Autodesk Fusion 360 part; units mm, degrees
(part 3 of 4)
  line L349 (-93.5315, -46.7348) -> (-93.5315, -40.9333)
  line L350 (-93.5315, -40.9333) -> (-94.3309, -40.9333)
  line L351 (-94.3309, -40.9333) -> (-94.3309, -37.8327)
  line L352 (-94.3309, -37.8327) -> (-93.5315, -37.8327)
  line L353 (-93.5315, -37.8327) -> (-93.5315, -36.8336)
  line L354 (-93.5315, -36.8336) -> (-79.5322, -36.8336)
  line L355 (-79.5322, -36.8336) -> (-79.5322, -37.8327)
  line L356 (-79.5322, -37.8327) -> (-78.7314, -37.8327)
  line L357 (-78.7314, -37.8327) -> (-78.7314, -40.9333)
  line L358 (-78.7314, -40.9333) -> (-79.5322, -40.9333)
  line L359 (-79.5322, -40.9333) -> (-79.5322, -46.7348)
  line L360 (-79.5322, -46.7348) -> (-78.7314, -46.7348)
  line L361 (-78.7314, -46.7348) -> (-78.7314, -49.8327)
  line L362 (-78.7314, -49.8327) -> (-79.5322, -49.8327)
  line L363 (-79.5322, -49.8327) -> (-79.5322, -50.833)
  line L364 (-98.5822, -50.833) -> (-112.5815, -50.833)
  line L365 (-112.5815, -50.833) -> (-112.5815, -49.8327)
  line L366 (-112.5815, -49.8327) -> (-113.3809, -49.8327)
  line L367 (-113.3809, -49.8327) -> (-113.3809, -46.7348)
  line L368 (-113.3809, -46.7348) -> (-112.5815, -46.7348)
  line L369 (-112.5815, -46.7348) -> (-112.5815, -40.9333)
  line L370 (-112.5815, -40.9333) -> (-113.3809, -40.9333)
  line L371 (-113.3809, -40.9333) -> (-113.3809, -37.8327)
  line L372 (-113.3809, -37.8327) -> (-112.5815, -37.8327)
  line L373 (-112.5815, -37.8327) -> (-112.5815, -36.8336)
  line L374 (-112.5815, -36.8336) -> (-98.5822, -36.8336)
  line L375 (-98.5822, -36.8336) -> (-98.5822, -37.8327)
  line L376 (-98.5822, -37.8327) -> (-97.7814, -37.8327)
  line L377 (-97.7814, -37.8327) -> (-97.7814, -40.9333)
  line L378 (-97.7814, -40.9333) -> (-98.5822, -40.9333)
  line L379 (-98.5822, -40.9333) -> (-98.5822, -46.7348)
  line L380 (-98.5822, -46.7348) -> (-97.7814, -46.7348)
  line L381 (-97.7814, -46.7348) -> (-97.7814, -49.8327)
  line L382 (-97.7814, -49.8327) -> (-98.5822, -49.8327)
  line L383 (-98.5822, -49.8327) -> (-98.5822, -50.833)
  line L384 (-227.17, -107.9831) -> (-241.169, -107.9831)
  line L385 (-241.169, -107.9831) -> (-241.169, -106.9826)
  line L386 (-241.169, -106.9826) -> (-241.97, -106.9826)
  line L387 (-241.97, -106.9826) -> (-241.97, -103.8834)
  line L388 (-241.97, -103.8834) -> (-241.169, -103.8834)
  line L389 (-241.169, -103.8834) -> (-241.169, -98.0834)
  line L390 (-241.169, -98.0834) -> (-241.97, -98.0834)
  line L391 (-241.97, -98.0834) -> (-241.97, -94.9828)
  line L392 (-241.97, -94.9828) -> (-241.169, -94.9828)
  line L393 (-241.169, -94.9828) -> (-241.169, -93.9838)
  line L394 (-241.169, -93.9838) -> (-227.17, -93.9838)
  line L395 (-227.17, -93.9838) -> (-227.17, -94.9828)
  line L396 (-227.17, -94.9828) -> (-226.369, -94.9828)
  line L397 (-226.369, -94.9828) -> (-226.369, -98.0834)
  line L398 (-226.369, -98.0834) -> (-227.17, -98.0834)
  line L399 (-227.17, -98.0834) -> (-227.17, -103.8834)
  line L400 (-227.17, -103.8834) -> (-226.369, -103.8834)
  line L401 (-226.369, -103.8834) -> (-226.369, -106.9826)
  line L402 (-226.369, -106.9826) -> (-227.17, -106.9826)
  line L403 (-227.17, -106.9826) -> (-227.17, -107.9831)
  line L404 (-193.832, -50.833) -> (-207.832, -50.833)
  line L405 (-207.832, -50.833) -> (-207.832, -49.8327)
  line L406 (-207.832, -49.8327) -> (-208.631, -49.8327)
  line L407 (-208.631, -49.8327) -> (-208.631, -46.7348)
  line L408 (-208.631, -46.7348) -> (-207.832, -46.7348)
  line L409 (-207.832, -46.7348) -> (-207.832, -40.9333)
  line L410 (-207.832, -40.9333) -> (-208.631, -40.9333)
  line L411 (-208.631, -40.9333) -> (-208.631, -37.8327)
  line L412 (-208.631, -37.8327) -> (-207.832, -37.8327)
  line L413 (-207.832, -37.8327) -> (-207.832, -36.8336)
  line L414 (-207.832, -36.8336) -> (-193.832, -36.8336)
  line L415 (-193.832, -36.8336) -> (-193.832, -37.8327)
  line L416 (-193.832, -37.8327) -> (-193.031, -37.8327)
  line L417 (-193.031, -37.8327) -> (-193.031, -40.9333)
  line L418 (-193.031, -40.9333) -> (-193.832, -40.9333)
  line L419 (-193.832, -40.9333) -> (-193.832, -46.7348)
  line L420 (-193.832, -46.7348) -> (-193.031, -46.7348)
  line L421 (-193.031, -46.7348) -> (-193.031, -49.8327)
  line L422 (-193.031, -49.8327) -> (-193.832, -49.8327)
  line L423 (-193.832, -49.8327) -> (-193.832, -50.833)
  line L424 (-65.2447, -88.9331) -> (-79.244, -88.9331)
  line L425 (-79.244, -88.9331) -> (-79.244, -87.9326)
  line L426 (-79.244, -87.9326) -> (-80.0448, -87.9326)
  line L427 (-80.0448, -87.9326) -> (-80.0448, -84.8334)
  line L428 (-80.0448, -84.8334) -> (-79.244, -84.8334)
  line L429 (-79.244, -84.8334) -> (-79.244, -79.0334)
  line L430 (-79.244, -79.0334) -> (-80.0448, -79.0334)
  line L431 (-80.0448, -79.0334) -> (-80.0448, -75.9328)
  line L432 (-80.0448, -75.9328) -> (-79.244, -75.9328)
  line L433 (-79.244, -75.9328) -> (-79.244, -74.9338)
  line L434 (-79.244, -74.9338) -> (-65.2447, -74.9338)
  line L435 (-65.2447, -74.9338) -> (-65.2447, -75.9328)
  line L436 (-65.2447, -75.9328) -> (-64.4439, -75.9328)
  line L437 (-64.4439, -75.9328) -> (-64.4439, -79.0334)
  line L438 (-64.4439, -79.0334) -> (-65.2447, -79.0334)
  line L439 (-65.2447, -79.0334) -> (-65.2447, -84.8334)
  line L440 (-65.2447, -84.8334) -> (-64.4439, -84.8334)
  line L441 (-64.4439, -84.8334) -> (-64.4439, -87.9326)
  line L442 (-64.4439, -87.9326) -> (-65.2447, -87.9326)
  line L443 (-65.2447, -87.9326) -> (-65.2447, -88.9331)
  line L444 (-198.595, -88.9331) -> (-212.594, -88.9331)
  line L445 (-212.594, -88.9331) -> (-212.594, -87.9326)
  line L446 (-212.594, -87.9326) -> (-213.395, -87.9326)
  line L447 (-213.395, -87.9326) -> (-213.395, -84.8334)
  line L448 (-213.395, -84.8334) -> (-212.594, -84.8334)
  line L449 (-212.594, -84.8334) -> (-212.594, -79.0334)
  line L450 (-212.594, -79.0334) -> (-213.395, -79.0334)
  line L451 (-213.395, -79.0334) -> (-213.395, -75.9328)
  line L452 (-213.395, -75.9328) -> (-212.594, -75.9328)
  line L453 (-212.594, -75.9328) -> (-212.594, -74.9338)
  line L454 (-212.594, -74.9338) -> (-198.595, -74.9338)
  line L455 (-198.595, -74.9338) -> (-198.595, -75.9328)
  line L456 (-198.595, -75.9328) -> (-197.794, -75.9328)
  line L457 (-197.794, -75.9328) -> (-197.794, -79.0334)
  line L458 (-197.794, -79.0334) -> (-198.595, -79.0334)
  line L459 (-198.595, -79.0334) -> (-198.595, -84.8334)
  line L460 (-198.595, -84.8334) -> (-197.794, -84.8334)
  line L461 (-197.794, -84.8334) -> (-197.794, -87.9326)
  line L462 (-197.794, -87.9326) -> (-198.595, -87.9326)
  line L463 (-198.595, -87.9326) -> (-198.595, -88.9331)
  line L464 (-222.407, -69.8831) -> (-236.407, -69.8831)
  line L465 (-236.407, -69.8831) -> (-236.407, -68.8826)
  line L466 (-236.407, -68.8826) -> (-237.206, -68.8826)
  line L467 (-237.206, -68.8826) -> (-237.206, -65.7834)
  line L468 (-237.206, -65.7834) -> (-236.407, -65.7834)
  line L469 (-236.407, -65.7834) -> (-236.407, -59.9834)
  line L470 (-236.407, -59.9834) -> (-237.206, -59.9834)
  line L471 (-237.206, -59.9834) -> (-237.206, -56.8828)
  line L472 (-237.206, -56.8828) -> (-236.407, -56.8828)
  line L473 (-236.407, -56.8828) -> (-236.407, -55.8838)
  line L474 (-236.407, -55.8838) -> (-222.407, -55.8838)
  line L475 (-222.407, -55.8838) -> (-222.407, -56.8828)
  line L476 (-222.407, -56.8828) -> (-221.606, -56.8828)
  line L477 (-221.606, -56.8828) -> (-221.606, -59.9834)
  line L478 (-221.606, -59.9834) -> (-222.407, -59.9834)
  line L479 (-222.407, -59.9834) -> (-222.407, -65.7834)
  line L480 (-222.407, -65.7834) -> (-221.606, -65.7834)
  line L481 (-221.606, -65.7834) -> (-221.606, -68.8826)
  line L482 (-221.606, -68.8826) -> (-222.407, -68.8826)
  line L483 (-222.407, -68.8826) -> (-222.407, -69.8831)
  line L484 (-122.395, -88.9331) -> (-136.394, -88.9331)
  line L485 (-136.394, -88.9331) -> (-136.394, -87.9326)
  line L486 (-136.394, -87.9326) -> (-137.195, -87.9326)
  line L487 (-137.195, -87.9326) -> (-137.195, -84.8334)
  line L488 (-137.195, -84.8334) -> (-136.394, -84.8334)
  line L489 (-136.394, -84.8334) -> (-136.394, -79.0334)
  line L490 (-136.394, -79.0334) -> (-137.195, -79.0334)
  line L491 (-137.195, -79.0334) -> (-137.195, -75.9328)
  line L492 (-137.195, -75.9328) -> (-136.394, -75.9328)
  line L493 (-136.394, -75.9328) -> (-136.394, -74.9338)
  line L494 (-136.394, -74.9338) -> (-122.395, -74.9338)
  line L495 (-122.395, -74.9338) -> (-122.395, -75.9328)
  line L496 (-122.395, -75.9328) -> (-121.594, -75.9328)
  line L497 (-121.594, -75.9328) -> (-121.594, -79.0334)
  line L498 (-121.594, -79.0334) -> (-122.395, -79.0334)
  line L499 (-122.395, -79.0334) -> (-122.395, -84.8334)
  line L500 (-122.395, -84.8334) -> (-121.594, -84.8334)
  line L501 (-121.594, -84.8334) -> (-121.594, -87.9326)
  line L502 (-121.594, -87.9326) -> (-122.395, -87.9326)
  line L503 (-122.395, -87.9326) -> (-122.395, -88.9331)
  line L504 (-89.0572, -69.8831) -> (-103.0565, -69.8831)
  line L505 (-103.0565, -69.8831) -> (-103.0565, -68.8826)
  line L506 (-103.0565, -68.8826) -> (-103.8559, -68.8826)
  line L507 (-103.8559, -68.8826) -> (-103.8559, -65.7834)
  line L508 (-103.8559, -65.7834) -> (-103.0565, -65.7834)
  line L509 (-103.0565, -65.7834) -> (-103.0565, -59.9834)
  line L510 (-103.0565, -59.9834) -> (-103.8559, -59.9834)
  line L511 (-103.8559, -59.9834) -> (-103.8559, -56.8828)
  line L512 (-103.8559, -56.8828) -> (-103.0565, -56.8828)
  line L513 (-103.0565, -56.8828) -> (-103.0565, -55.8838)
  line L514 (-103.0565, -55.8838) -> (-89.0572, -55.8838)
  line L515 (-89.0572, -55.8838) -> (-89.0572, -56.8828)
  line L516 (-89.0572, -56.8828) -> (-88.2564, -56.8828)
  line L517 (-88.2564, -56.8828) -> (-88.2564, -59.9834)
  line L518 (-88.2564, -59.9834) -> (-89.0572, -59.9834)
  line L519 (-89.0572, -59.9834) -> (-89.0572, -65.7834)
  line L520 (-89.0572, -65.7834) -> (-88.2564, -65.7834)
  line L521 (-88.2564, -65.7834) -> (-88.2564, -68.8826)
  line L522 (-88.2564, -68.8826) -> (-89.0572, -68.8826)
  line L523 (-89.0572, -68.8826) -> (-89.0572, -69.8831)
  line L524 (-160.495, -88.9331) -> (-174.494, -88.9331)
  line L525 (-174.494, -88.9331) -> (-174.494, -87.9326)
  line L526 (-174.494, -87.9326) -> (-175.295, -87.9326)
  line L527 (-175.295, -87.9326) -> (-175.295, -84.8334)
  line L528 (-175.295, -84.8334) -> (-174.494, -84.8334)
  line L529 (-174.494, -84.8334) -> (-174.494, -79.0334)
  line L530 (-174.494, -79.0334) -> (-175.295, -79.0334)
  line L531 (-175.295, -79.0334) -> (-175.295, -75.9328)
  line L532 (-175.295, -75.9328) -> (-174.494, -75.9328)
  line L533 (-174.494, -75.9328) -> (-174.494, -74.9338)
  line L534 (-174.494, -74.9338) -> (-160.495, -74.9338)
  line L535 (-160.495, -74.9338) -> (-160.495, -75.9328)
  line L536 (-160.495, -75.9328) -> (-159.694, -75.9328)
  line L537 (-159.694, -75.9328) -> (-159.694, -79.0334)
  line L538 (-159.694, -79.0334) -> (-160.495, -79.0334)
  line L539 (-160.495, -79.0334) -> (-160.495, -84.8334)
  line L540 (-160.495, -84.8334) -> (-159.694, -84.8334)
  line L541 (-159.694, -84.8334) -> (-159.694, -87.9326)
  line L542 (-159.694, -87.9326) -> (-160.495, -87.9326)
  line L543 (-160.495, -87.9326) -> (-160.495, -88.9331)
  line L544 (-139.062, -31.7831) -> (-153.063, -31.7831)
  line L545 (-153.063, -31.7831) -> (-153.063, -30.7827)
  line L546 (-153.063, -30.7827) -> (-153.862, -30.7827)
  line L547 (-153.862, -30.7827) -> (-153.862, -27.6848)
  line L548 (-153.862, -27.6848) -> (-153.063, -27.6848)
  line L549 (-153.063, -27.6848) -> (-153.063, -27.0826)
  line L550 (-153.063, -27.0826) -> (-192.687, -27.0826)
  line L551 (-192.687, -27.0826) -> (-192.687, -30.3128)
  line L552 (-192.687, -30.3128) -> (-194.412, -30.3128)
  line L553 (-194.412, -30.3128) -> (-194.412, -31.2347)
  line L554 (-194.412, -31.2347) -> (-197.713, -31.2347)
  line L555 (-197.713, -31.2347) -> (-197.713, -30.3128)
  line L556 (-197.713, -30.3128) -> (-199.438, -30.3128)
  line L557 (-199.438, -30.3128) -> (-199.438, -27.0826)
  line L558 (-199.438, -27.0826) -> (-200.262, -27.0826)
  line L559 (-200.262, -27.0826) -> (-200.262, -24.2838)
  line L560 (-200.262, -24.2838) -> (-199.438, -24.2838)
  line L561 (-199.438, -24.2838) -> (-199.438, -18.0138)
  line L562 (-199.438, -18.0138) -> (-197.713, -18.0138)
  line L563 (-197.713, -18.0138) -> (-197.713, -17.0326)
  line L564 (-197.713, -17.0326) -> (-194.412, -17.0326)
  line L565 (-194.412, -17.0326) -> (-194.412, -18.0138)
  line L566 (-194.412, -18.0138) -> (-192.687, -18.0138)
  line L567 (-192.687, -18.0138) -> (-192.687, -22.4841)
  line L568 (-192.687, -22.4841) -> (-153.063, -22.4841)
  line L569 (-153.063, -22.4841) -> (-153.063, -21.8833)
  line L570 (-153.063, -21.8833) -> (-153.862, -21.8833)
  line L571 (-153.862, -21.8833) -> (-153.862, -18.7827)
  line L572 (-153.862, -18.7827) -> (-153.063, -18.7827)
  line L573 (-153.063, -18.7827) -> (-153.063, -17.7836)
  line L574 (-153.063, -17.7836) -> (-139.062, -17.7836)
  line L575 (-139.062, -17.7836) -> (-139.062, -18.7827)
  line L576 (-139.062, -18.7827) -> (-138.263, -18.7827)
  line L577 (-138.263, -18.7827) -> (-138.263, -21.8833)
  line L578 (-138.263, -21.8833) -> (-139.062, -21.8833)
  line L579 (-139.062, -21.8833) -> (-139.062, -22.4841)
  line L580 (-139.062, -22.4841) -> (-99.4381, -22.4841)
  line L581 (-99.4381, -22.4841) -> (-99.4381, -18.0138)
  line L582 (-99.4381, -18.0138) -> (-97.7126, -18.0138)
  line L583 (-97.7126, -18.0138) -> (-97.7126, -17.0326)
  line L584 (-97.7126, -17.0326) -> (-94.412, -17.0326)
  line L585 (-94.412, -17.0326) -> (-94.412, -18.0138)
  line L586 (-94.412, -18.0138) -> (-92.687, -18.0138)
  line L587 (-92.687, -18.0138) -> (-92.687, -24.2838)
  line L588 (-92.687, -24.2838) -> (-91.8629, -24.2838)
  line L589 (-91.8629, -24.2838) -> (-91.8629, -27.0826)
  line L590 (-91.8629, -27.0826) -> (-92.687, -27.0826)
  line L591 (-92.687, -27.0826) -> (-92.687, -30.3128)
  line L592 (-92.687, -30.3128) -> (-94.412, -30.3128)
  line L593 (-94.412, -30.3128) -> (-94.412, -31.2347)
  line L594 (-94.412, -31.2347) -> (-97.7126, -31.2347)
  line L595 (-97.7126, -31.2347) -> (-97.7126, -30.3128)
  line L596 (-97.7126, -30.3128) -> (-99.4381, -30.3128)
  line L597 (-99.4381, -30.3128) -> (-99.4381, -27.0826)
  line L598 (-99.4381, -27.0826) -> (-139.062, -27.0826)
  line L599 (-139.062, -27.0826) -> (-139.062, -27.6848)
  line L600 (-139.062, -27.6848) -> (-138.263, -27.6848)
  line L601 (-138.263, -27.6848) -> (-138.263, -30.7827)
  line L602 (-138.263, -30.7827) -> (-139.062, -30.7827)
  line L603 (-139.062, -30.7827) -> (-139.062, -31.7831)
  line L604 (-272.412, -69.8831) -> (-286.413, -69.8831)
  line L605 (-286.413, -69.8831) -> (-286.413, -68.8826)
  line L606 (-286.413, -68.8826) -> (-287.212, -68.8826)
  line L607 (-287.212, -68.8826) -> (-287.212, -65.7834)
  line L608 (-287.212, -65.7834) -> (-286.413, -65.7834)
  line L609 (-286.413, -65.7834) -> (-286.413, -65.1826)
  line L610 (-286.413, -65.1826) -> (-287.937, -65.1826)
  line L611 (-287.937, -65.1826) -> (-287.937, -68.4127)
  line L612 (-287.937, -68.4127) -> (-289.662, -68.4127)
  line L613 (-289.662, -68.4127) -> (-289.662, -69.3334)
  line L614 (-289.662, -69.3334) -> (-292.963, -69.3334)
  line L615 (-292.963, -69.3334) -> (-292.963, -68.4127)
  line L616 (-292.963, -68.4127) -> (-294.688, -68.4127)
  line L617 (-294.688, -68.4127) -> (-294.688, -65.1826)
  line L618 (-294.688, -65.1826) -> (-295.512, -65.1826)
  line L619 (-295.512, -65.1826) -> (-295.512, -62.3837)
  line L620 (-295.512, -62.3837) -> (-294.688, -62.3837)
  line L621 (-294.688, -62.3837) -> (-294.688, -56.1138)
  line L622 (-294.688, -56.1138) -> (-292.963, -56.1138)
  line L623 (-292.963, -56.1138) -> (-292.963, -55.1327)
  line L624 (-292.963, -55.1327) -> (-289.662, -55.1327)
  line L625 (-289.662, -55.1327) -> (-289.662, -56.1138)
  line L626 (-289.662, -56.1138) -> (-287.937, -56.1138)
  line L627 (-287.937, -56.1138) -> (-287.937, -60.5828)
  line L628 (-287.937, -60.5828) -> (-286.413, -60.5828)
  line L629 (-286.413, -60.5828) -> (-286.413, -59.9834)
  line L630 (-286.413, -59.9834) -> (-287.212, -59.9834)
  line L631 (-287.212, -59.9834) -> (-287.212, -56.8828)
  line L632 (-287.212, -56.8828) -> (-286.413, -56.8828)
  line L633 (-286.413, -56.8828) -> (-286.413, -55.8838)
  line L634 (-286.413, -55.8838) -> (-272.412, -55.8838)
  line L635 (-272.412, -55.8838) -> (-272.412, -56.8828)
  line L636 (-272.412, -56.8828) -> (-271.611, -56.8828)
  line L637 (-271.611, -56.8828) -> (-271.611, -59.9834)
  line L638 (-271.611, -59.9834) -> (-272.412, -59.9834)
  line L639 (-272.412, -59.9834) -> (-272.412, -60.5828)
  line L640 (-272.412, -60.5828) -> (-270.888, -60.5828)
  line L641 (-270.888, -60.5828) -> (-270.888, -56.1138)
  line L642 (-270.888, -56.1138) -> (-269.161, -56.1138)
  line L643 (-269.161, -56.1138) -> (-269.161, -55.1327)
  line L644 (-269.161, -55.1327) -> (-265.862, -55.1327)
  line L645 (-265.862, -55.1327) -> (-265.862, -56.1138)
  line L646 (-265.862, -56.1138) -> (-264.137, -56.1138)
  line L647 (-264.137, -56.1138) -> (-264.137, -62.3837)
  line L648 (-264.137, -62.3837) -> (-263.313, -62.3837)
  line L649 (-263.313, -62.3837) -> (-263.313, -65.1826)
  line L650 (-263.313, -65.1826) -> (-264.137, -65.1826)
  line L651 (-264.137, -65.1826) -> (-264.137, -68.4127)
  line L652 (-264.137, -68.4127) -> (-265.862, -68.4127)
  line L653 (-265.862, -68.4127) -> (-265.862, -69.3334)
  line L654 (-265.862, -69.3334) -> (-269.161, -69.3334)
  line L655 (-269.161, -69.3334) -> (-269.161, -68.4127)
  line L656 (-269.161, -68.4127) -> (-270.888, -68.4127)
  line L657 (-270.888, -68.4127) -> (-270.888, -65.1826)
  line L658 (-270.888, -65.1826) -> (-272.412, -65.1826)
  line L659 (-272.412, -65.1826) -> (-272.412, -65.7834)
  line L660 (-272.412, -65.7834) -> (-271.611, -65.7834)
  line L661 (-271.611, -65.7834) -> (-271.611, -68.8826)
  line L662 (-271.611, -68.8826) -> (-272.412, -68.8826)
  line L663 (-272.412, -68.8826) -> (-272.412, -69.8831)
  line L664 (-274.795, -107.9831) -> (-288.794, -107.9831)
  line L665 (-288.794, -107.9831) -> (-288.794, -106.9826)
  line L666 (-288.794, -106.9826) -> (-289.595, -106.9826)
  line L667 (-289.595, -106.9826) -> (-289.595, -103.8834)
  line L668 (-289.595, -103.8834) -> (-288.794, -103.8834)
  line L669 (-288.794, -103.8834) -> (-288.794, -103.2826)
  line L670 (-288.794, -103.2826) -> (-290.32, -103.2826)
  line L671 (-290.32, -103.2826) -> (-290.32, -106.5127)
  line L672 (-290.32, -106.5127) -> (-292.045, -106.5127)
  line L673 (-292.045, -106.5127) -> (-292.045, -107.4348)
  line L674 (-292.045, -107.4348) -> (-295.344, -107.4348)
  line L675 (-295.344, -107.4348) -> (-295.344, -106.5127)
  line L676 (-295.344, -106.5127) -> (-297.069, -106.5127)
  line L677 (-297.069, -106.5127) -> (-297.069, -103.2826)
  line L678 (-297.069, -103.2826) -> (-297.895, -103.2826)
  line L679 (-297.895, -103.2826) -> (-297.895, -100.4837)
  line L680 (-297.895, -100.4837) -> (-297.069, -100.4837)
  line L681 (-297.069, -100.4837) -> (-297.069, -94.2138)
  line L682 (-297.069, -94.2138) -> (-295.344, -94.2138)
  line L683 (-295.344, -94.2138) -> (-295.344, -93.2327)
  line L684 (-295.344, -93.2327) -> (-292.045, -93.2327)
  line L685 (-292.045, -93.2327) -> (-292.045, -94.2138)
  line L686 (-292.045, -94.2138) -> (-290.32, -94.2138)
  line L687 (-290.32, -94.2138) -> (-290.32, -98.6828)
  line L688 (-290.32, -98.6828) -> (-288.794, -98.6828)
  line L689 (-288.794, -98.6828) -> (-288.794, -98.0834)
  line L690 (-288.794, -98.0834) -> (-289.595, -98.0834)
  line L691 (-289.595, -98.0834) -> (-289.595, -94.9828)
  line L692 (-289.595, -94.9828) -> (-288.794, -94.9828)
  line L693 (-288.794, -94.9828) -> (-288.794, -93.9838)
  line L694 (-288.794, -93.9838) -> (-274.795, -93.9838)
  line L695 (-274.795, -93.9838) -> (-274.795, -94.9828)
  line L696 (-274.795, -94.9828) -> (-273.994, -94.9828)
  line L697 (-273.994, -94.9828) -> (-273.994, -98.0834)
  line L698 (-273.994, -98.0834) -> (-274.795, -98.0834)
  line L699 (-274.795, -98.0834) -> (-274.795, -98.6828)
  line L700 (-274.795, -98.6828) -> (-273.269, -98.6828)
  line L701 (-273.269, -98.6828) -> (-273.269, -94.2138)
  line L702 (-273.269, -94.2138) -> (-271.544, -94.2138)
  line L703 (-271.544, -94.2138) -> (-271.544, -93.2327)
  line L704 (-271.544, -93.2327) -> (-268.243, -93.2327)
  line L705 (-268.243, -93.2327) -> (-268.243, -94.2138)
  line L706 (-268.243, -94.2138) -> (-266.52, -94.2138)
  line L707 (-266.52, -94.2138) -> (-266.52, -100.4837)
  line L708 (-266.52, -100.4837) -> (-265.694, -100.4837)
  line L709 (-265.694, -100.4837) -> (-265.694, -103.2826)
  line L710 (-265.694, -103.2826) -> (-266.52, -103.2826)
  line L711 (-266.52, -103.2826) -> (-266.52, -106.5127)
  line L712 (-266.52, -106.5127) -> (-268.243, -106.5127)
  line L713 (-268.243, -106.5127) -> (-268.243, -107.4348)
  line L714 (-268.243, -107.4348) -> (-271.544, -107.4348)
  line L715 (-271.544, -107.4348) -> (-271.544, -106.5127)
  line L716 (-271.544, -106.5127) -> (-273.269, -106.5127)
  line L717 (-273.269, -106.5127) -> (-273.269, -103.2826)
  line L718 (-273.269, -103.2826) -> (-274.795, -103.2826)
  line L719 (-274.795, -103.2826) -> (-274.795, -103.8834)
  line L720 (-274.795, -103.8834) -> (-273.994, -103.8834)
  line L721 (-273.994, -103.8834) -> (-273.994, -106.9826)
  line L722 (-273.994, -106.9826) -> (-274.795, -106.9826)
  line L723 (-274.795, -106.9826) -> (-274.795, -107.9831)
  line L724 (-281.937, -31.7831) -> (-295.938, -31.7831)
  line L725 (-295.938, -31.7831) -> (-295.938, -30.7827)
  line L726 (-295.938, -30.7827) -> (-296.737, -30.7827)
  line L727 (-296.737, -30.7827) -> (-296.737, -27.6848)
  line L728 (-296.737, -27.6848) -> (-295.938, -27.6848)
  line L729 (-295.938, -27.6848) -> (-295.938, -21.8833)
  line L730 (-295.938, -21.8833) -> (-296.737, -21.8833)
  line L731 (-296.737, -21.8833) -> (-296.737, -18.7827)
  line L732 (-296.737, -18.7827) -> (-295.938, -18.7827)
  line L733 (-295.938, -18.7827) -> (-295.938, -17.7836)
  line L734 (-295.938, -17.7836) -> (-281.937, -17.7836)
  line L735 (-281.937, -17.7836) -> (-281.937, -18.7827)
  line L736 (-281.937, -18.7827) -> (-281.138, -18.7827)
  line L737 (-281.138, -18.7827) -> (-281.138, -21.8833)
  line L738 (-281.138, -21.8833) -> (-281.937, -21.8833)
  line L739 (-281.937, -21.8833) -> (-281.937, -27.6848)
  line L740 (-281.937, -27.6848) -> (-281.138, -27.6848)
  line L741 (-281.138, -27.6848) -> (-281.138, -30.7827)
  line L742 (-281.138, -30.7827) -> (-281.937, -30.7827)
  line L743 (-281.937, -30.7827) -> (-281.937, -31.7831)
  line L744 (-184.307, -69.8831) -> (-198.307, -69.8831)
  line L745 (-198.307, -69.8831) -> (-198.307, -68.8826)
  line L746 (-198.307, -68.8826) -> (-199.106, -68.8826)
  line L747 (-199.106, -68.8826) -> (-199.106, -65.7834)
  line L748 (-199.106, -65.7834) -> (-198.307, -65.7834)
  line L749 (-198.307, -65.7834) -> (-198.307, -59.9834)
  line L750 (-198.307, -59.9834) -> (-199.106, -59.9834)
  line L751 (-199.106, -59.9834) -> (-199.106, -56.8828)
  line L752 (-199.106, -56.8828) -> (-198.307, -56.8828)
  line L753 (-198.307, -56.8828) -> (-198.307, -55.8838)
  line L754 (-198.307, -55.8838) -> (-184.307, -55.8838)
  line L755 (-184.307, -55.8838) -> (-184.307, -56.8828)
  line L756 (-184.307, -56.8828) -> (-183.506, -56.8828)
  line L757 (-183.506, -56.8828) -> (-183.506, -59.9834)
  line L758 (-183.506, -59.9834) -> (-184.307, -59.9834)
  line L759 (-184.307, -59.9834) -> (-184.307, -65.7834)
  line L760 (-184.307, -65.7834) -> (-183.506, -65.7834)
  line L761 (-183.506, -65.7834) -> (-183.506, -68.8826)
  line L762 (-183.506, -68.8826) -> (-184.307, -68.8826)
  line L763 (-184.307, -68.8826) -> (-184.307, -69.8831)
  line L764 (-217.645, -88.9331) -> (-231.644, -88.9331)
  line L765 (-231.644, -88.9331) -> (-231.644, -87.9326)
  line L766 (-231.644, -87.9326) -> (-232.445, -87.9326)
  line L767 (-232.445, -87.9326) -> (-232.445, -84.8334)
  line L768 (-232.445, -84.8334) -> (-231.644, -84.8334)
  line L769 (-231.644, -84.8334) -> (-231.644, -79.0334)
  line L770 (-231.644, -79.0334) -> (-232.445, -79.0334)
  line L771 (-232.445, -79.0334) -> (-232.445, -75.9328)
  line L772 (-232.445, -75.9328) -> (-231.644, -75.9328)
  line L773 (-231.644, -75.9328) -> (-231.644, -74.9338)
  line L774 (-231.644, -74.9338) -> (-217.645, -74.9338)
  line L775 (-217.645, -74.9338) -> (-217.645, -75.9328)
  line L776 (-217.645, -75.9328) -> (-216.844, -75.9328)
  line L777 (-216.844, -75.9328) -> (-216.844, -79.0334)
  line L778 (-216.844, -79.0334) -> (-217.645, -79.0334)
  line L779 (-217.645, -79.0334) -> (-217.645, -84.8334)
  line L780 (-217.645, -84.8334) -> (-216.844, -84.8334)
  line L781 (-216.844, -84.8334) -> (-216.844, -87.9326)
  line L782 (-216.844, -87.9326) -> (-217.645, -87.9326)
  line L783 (-217.645, -87.9326) -> (-217.645, -88.9331)
  line L784 (-165.257, -69.8831) -> (-179.257, -69.8831)
  line L785 (-179.257, -69.8831) -> (-179.257, -68.8826)
  line L786 (-179.257, -68.8826) -> (-180.056, -68.8826)
  line L787 (-180.056, -68.8826) -> (-180.056, -65.7834)
  line L788 (-180.056, -65.7834) -> (-179.257, -65.7834)
  line L789 (-179.257, -65.7834) -> (-179.257, -59.9834)
  line L790 (-179.257, -59.9834) -> (-180.056, -59.9834)
  line L791 (-180.056, -59.9834) -> (-180.056, -56.8828)
  line L792 (-180.056, -56.8828) -> (-179.257, -56.8828)
  line L793 (-179.257, -56.8828) -> (-179.257, -55.8838)
  line L794 (-179.257, -55.8838) -> (-165.257, -55.8838)
  line L795 (-165.257, -55.8838) -> (-165.257, -56.8828)
  line L796 (-165.257, -56.8828) -> (-164.456, -56.8828)
  line L797 (-164.456, -56.8828) -> (-164.456, -59.9834)
  line L798 (-164.456, -59.9834) -> (-165.257, -59.9834)
  line L799 (-165.257, -59.9834) -> (-165.257, -65.7834)
  line L800 (-165.257, -65.7834) -> (-164.456, -65.7834)
  line L801 (-164.456, -65.7834) -> (-164.456, -68.8826)
  line L802 (-164.456, -68.8826) -> (-165.257, -68.8826)
  line L803 (-165.257, -68.8826) -> (-165.257, -69.8831)
  line L804 (-103.3447, -88.9331) -> (-117.344, -88.9331)
  line L805 (-117.344, -88.9331) -> (-117.344, -87.9326)
  line L806 (-117.344, -87.9326) -> (-118.145, -87.9326)
  line L807 (-118.145, -87.9326) -> (-118.145, -84.8334)
  line L808 (-118.145, -84.8334) -> (-117.344, -84.8334)
  line L809 (-117.344, -84.8334) -> (-117.344, -79.0334)
  line L810 (-117.344, -79.0334) -> (-118.145, -79.0334)
  line L811 (-118.145, -79.0334) -> (-118.145, -75.9328)
  line L812 (-118.145, -75.9328) -> (-117.344, -75.9328)
  line L813 (-117.344, -75.9328) -> (-117.344, -74.9338)
  line L814 (-117.344, -74.9338) -> (-103.3447, -74.9338)
  line L815 (-103.3447, -74.9338) -> (-103.3447, -75.9328)
  line L816 (-103.3447, -75.9328) -> (-102.5439, -75.9328)
  line L817 (-102.5439, -75.9328) -> (-102.5439, -79.0334)
  line L818 (-102.5439, -79.0334) -> (-103.3447, -79.0334)
  line L819 (-103.3447, -79.0334) -> (-103.3447, -84.8334)
  line L820 (-103.3447, -84.8334) -> (-102.5439, -84.8334)
  line L821 (-102.5439, -84.8334) -> (-102.5439, -87.9326)
  line L822 (-102.5439, -87.9326) -> (-103.3447, -87.9326)
  line L823 (-103.3447, -87.9326) -> (-103.3447, -88.9331)
  line L824 (-70.0072, -69.8831) -> (-84.0065, -69.8831)
  line L825 (-84.0065, -69.8831) -> (-84.0065, -68.8826)
  line L826 (-84.0065, -68.8826) -> (-84.8059, -68.8826)
  line L827 (-84.8059, -68.8826) -> (-84.8059, -65.7834)
  line L828 (-84.8059, -65.7834) -> (-84.0065, -65.7834)
  line L829 (-84.0065, -65.7834) -> (-84.0065, -59.9834)
  line L830 (-84.0065, -59.9834) -> (-84.8059, -59.9834)
  line L831 (-84.8059, -59.9834) -> (-84.8059, -56.8828)
  line L832 (-84.8059, -56.8828) -> (-84.0065, -56.8828)
  line L833 (-84.0065, -56.8828) -> (-84.0065, -55.8838)
  line L834 (-84.0065, -55.8838) -> (-70.0072, -55.8838)
  line L835 (-70.0072, -55.8838) -> (-70.0072, -56.8828)
  line L836 (-70.0072, -56.8828) -> (-69.2064, -56.8828)
  line L837 (-69.2064, -56.8828) -> (-69.2064, -59.9834)
  line L838 (-69.2064, -59.9834) -> (-70.0072, -59.9834)
  line L839 (-70.0072, -59.9834) -> (-70.0072, -65.7834)
  line L840 (-70.0072, -65.7834) -> (-69.2064, -65.7834)
  line L841 (-69.2064, -65.7834) -> (-69.2064, -68.8826)
  line L842 (-69.2064, -68.8826) -> (-70.0072, -68.8826)
  line L843 (-70.0072, -68.8826) -> (-70.0072, -69.8831)
  line L844 (-108.1072, -69.8831) -> (-122.107, -69.8831)
  line L845 (-122.107, -69.8831) -> (-122.107, -68.8826)
  line L846 (-122.107, -68.8826) -> (-122.906, -68.8826)
  line L847 (-122.906, -68.8826) -> (-122.906, -65.7834)
  line L848 (-122.906, -65.7834) -> (-122.107, -65.7834)
  line L849 (-122.107, -65.7834) -> (-122.107, -59.9834)
  line L850 (-122.107, -59.9834) -> (-122.906, -59.9834)
  line L851 (-122.906, -59.9834) -> (-122.906, -56.8828)
  line L852 (-122.906, -56.8828) -> (-122.107, -56.8828)
  line L853 (-122.107, -56.8828) -> (-122.107, -55.8838)
  line L854 (-122.107, -55.8838) -> (-108.1072, -55.8838)
  line L855 (-108.1072, -55.8838) -> (-108.1072, -56.8828)
  line L856 (-108.1072, -56.8828) -> (-107.3064, -56.8828)
  line L857 (-107.3064, -56.8828) -> (-107.3064, -59.9834)
  line L858 (-107.3064, -59.9834) -> (-108.1072, -59.9834)
  line L859 (-108.1072, -59.9834) -> (-108.1072, -65.7834)
  line L860 (-108.1072, -65.7834) -> (-107.3064, -65.7834)
  line L861 (-107.3064, -65.7834) -> (-107.3064, -68.8826)
  line L862 (-107.3064, -68.8826) -> (-108.1072, -68.8826)
  line L863 (-108.1072, -68.8826) -> (-108.1072, -69.8831)
  line L864 (-20.0009, -31.7831) -> (-34.0004, -31.7831)
  line L865 (-34.0004, -31.7831) -> (-34.0004, -30.7827)
  line L866 (-34.0004, -30.7827) -> (-34.801, -30.7827)
  line L867 (-34.801, -30.7827) -> (-34.801, -27.6848)
  line L868 (-34.801, -27.6848) -> (-34.0004, -27.6848)
  line L869 (-34.0004, -27.6848) -> (-34.0004, -21.8833)
  line L870 (-34.0004, -21.8833) -> (-34.801, -21.8833)
  line L871 (-34.801, -21.8833) -> (-34.801, -18.7827)
  line L872 (-34.801, -18.7827) -> (-34.0004, -18.7827)
  line L873 (-34.0004, -18.7827) -> (-34.0004, -17.7836)
  line L874 (-34.0004, -17.7836) -> (-20.0009, -17.7836)
  line L875 (-20.0009, -17.7836) -> (-20.0009, -18.7827)
  line L876 (-20.0009, -18.7827) -> (-19.2003, -18.7827)
  line L877 (-19.2003, -18.7827) -> (-19.2003, -21.8833)
  line L878 (-19.2003, -21.8833) -> (-20.0009, -21.8833)
  line L879 (-20.0009, -21.8833) -> (-20.0009, -27.6848)
  line L880 (-20.0009, -27.6848) -> (-19.2003, -27.6848)
  line L881 (-19.2003, -27.6848) -> (-19.2003, -30.7827)
  line L882 (-19.2003, -30.7827) -> (-20.0009, -30.7827)
  line L883 (-20.0009, -30.7827) -> (-20.0009, -31.7831)
  line L884 (-84.2947, -88.9331) -> (-98.294, -88.9331)
  line L885 (-98.294, -88.9331) -> (-98.294, -87.9326)
  line L886 (-98.294, -87.9326) -> (-99.0948, -87.9326)
  line L887 (-99.0948, -87.9326) -> (-99.0948, -84.8334)
  line L888 (-99.0948, -84.8334) -> (-98.294, -84.8334)
  line L889 (-98.294, -84.8334) -> (-98.294, -79.0334)
  line L890 (-98.294, -79.0334) -> (-99.0948, -79.0334)
  line L891 (-99.0948, -79.0334) -> (-99.0948, -75.9328)
  line L892 (-99.0948, -75.9328) -> (-98.294, -75.9328)
  line L893 (-98.294, -75.9328) -> (-98.294, -74.9338)
  line L894 (-98.294, -74.9338) -> (-84.2947, -74.9338)
  line L895 (-84.2947, -74.9338) -> (-84.2947, -75.9328)
  line L896 (-84.2947, -75.9328) -> (-83.4939, -75.9328)
  line L897 (-83.4939, -75.9328) -> (-83.4939, -79.0334)
  line L898 (-83.4939, -79.0334) -> (-84.2947, -79.0334)
  line L899 (-84.2947, -79.0334) -> (-84.2947, -84.8334)
  line L900 (-84.2947, -84.8334) -> (-83.4939, -84.8334)
  line L901 (-83.4939, -84.8334) -> (-83.4939, -87.9326)
  line L902 (-83.4939, -87.9326) -> (-84.2947, -87.9326)
  line L903 (-84.2947, -87.9326) -> (-84.2947, -88.9331)
  line L904 (-46.1947, -88.9331) -> (-60.194, -88.9331)
  line L905 (-60.194, -88.9331) -> (-60.194, -87.9326)
  line L906 (-60.194, -87.9326) -> (-60.9948, -87.9326)
  line L907 (-60.9948, -87.9326) -> (-60.9948, -84.8334)
  line L908 (-60.9948, -84.8334) -> (-60.194, -84.8334)
  line L909 (-60.194, -84.8334) -> (-60.194, -79.0334)
  line L910 (-60.194, -79.0334) -> (-60.9948, -79.0334)
  line L911 (-60.9948, -79.0334) -> (-60.9948, -75.9328)
  line L912 (-60.9948, -75.9328) -> (-60.194, -75.9328)
  line L913 (-60.194, -75.9328) -> (-60.194, -74.9338)
  line L914 (-60.194, -74.9338) -> (-46.1947, -74.9338)
  line L915 (-46.1947, -74.9338) -> (-46.1947, -75.9328)
  line L916 (-46.1947, -75.9328) -> (-45.394, -75.9328)
  line L917 (-45.394, -75.9328) -> (-45.394, -79.0334)
  line L918 (-45.394, -79.0334) -> (-46.1947, -79.0334)
  line L919 (-46.1947, -79.0334) -> (-46.1947, -84.8334)
  line L920 (-46.1947, -84.8334) -> (-45.394, -84.8334)
  line L921 (-45.394, -84.8334) -> (-45.394, -87.9326)
  line L922 (-45.394, -87.9326) -> (-46.1947, -87.9326)
  line L923 (-46.1947, -87.9326) -> (-46.1947, -88.9331)
  line L924 (-212.882, -50.833) -> (-226.882, -50.833)
  line L925 (-226.882, -50.833) -> (-226.882, -49.8327)
  line L926 (-226.882, -49.8327) -> (-227.681, -49.8327)
  line L927 (-227.681, -49.8327) -> (-227.681, -46.7348)
  line L928 (-227.681, -46.7348) -> (-226.882, -46.7348)
  line L929 (-226.882, -46.7348) -> (-226.882, -40.9333)
  line L930 (-226.882, -40.9333) -> (-227.681, -40.9333)
  line L931 (-227.681, -40.9333) -> (-227.681, -37.8327)
  line L932 (-227.681, -37.8327) -> (-226.882, -37.8327)
  line L933 (-226.882, -37.8327) -> (-226.882, -36.8336)
  line L934 (-226.882, -36.8336) -> (-212.882, -36.8336)
  line L935 (-212.882, -36.8336) -> (-212.882, -37.8327)
  line L936 (-212.882, -37.8327) -> (-212.081, -37.8327)
  line L937 (-212.081, -37.8327) -> (-212.081, -40.9333)
  line L938 (-212.081, -40.9333) -> (-212.882, -40.9333)
  line L939 (-212.882, -40.9333) -> (-212.882, -46.7348)
  line L940 (-212.882, -46.7348) -> (-212.081, -46.7348)
  line L941 (-212.081, -46.7348) -> (-212.081, -49.8327)
  line L942 (-212.081, -49.8327) -> (-212.882, -49.8327)
  line L943 (-212.882, -49.8327) -> (-212.882, -50.833)
  line L944 (-136.682, -50.833) -> (-150.682, -50.833)
  line L945 (-150.682, -50.833) -> (-150.682, -49.8327)
  line L946 (-150.682, -49.8327) -> (-151.481, -49.8327)
  line L947 (-151.481, -49.8327) -> (-151.481, -46.7348)
  line L948 (-151.481, -46.7348) -> (-150.682, -46.7348)
  line L949 (-150.682, -46.7348) -> (-150.682, -40.9333)
  line L950 (-150.682, -40.9333) -> (-151.481, -40.9333)
  line L951 (-151.481, -40.9333) -> (-151.481, -37.8327)
  line L952 (-151.481, -37.8327) -> (-150.682, -37.8327)
  line L953 (-150.682, -37.8327) -> (-150.682, -36.8336)
  line L954 (-150.682, -36.8336) -> (-136.682, -36.8336)
  line L955 (-136.682, -36.8336) -> (-136.682, -37.8327)
  line L956 (-136.682, -37.8327) -> (-135.881, -37.8327)
  line L957 (-135.881, -37.8327) -> (-135.881, -40.9333)
  line L958 (-135.881, -40.9333) -> (-136.682, -40.9333)
  line L959 (-136.682, -40.9333) -> (-136.682, -46.7348)
  line L960 (-136.682, -46.7348) -> (-135.881, -46.7348)
  line L961 (-135.881, -46.7348) -> (-135.881, -49.8327)
  line L962 (-135.881, -49.8327) -> (-136.682, -49.8327)
  line L963 (-136.682, -49.8327) -> (-136.682, -50.833)
  line L964 (-117.632, -50.833) -> (-131.632, -50.833)
  line L965 (-131.632, -50.833) -> (-131.632, -49.8327)
  line L966 (-131.632, -49.8327) -> (-132.431, -49.8327)
  line L967 (-132.431, -49.8327) -> (-132.431, -46.7348)
  line L968 (-132.431, -46.7348) -> (-131.632, -46.7348)
  line L969 (-131.632, -46.7348) -> (-131.632, -40.9333)
  line L970 (-131.632, -40.9333) -> (-132.431, -40.9333)
  line L971 (-132.431, -40.9333) -> (-132.431, -37.8327)
  line L972 (-132.431, -37.8327) -> (-131.632, -37.8327)
  line L973 (-131.632, -37.8327) -> (-131.632, -36.8336)
  line L974 (-131.632, -36.8336) -> (-117.632, -36.8336)
  line L975 (-117.632, -36.8336) -> (-117.632, -37.8327)
  line L976 (-117.632, -37.8327) -> (-116.831, -37.8327)
  line L977 (-116.831, -37.8327) -> (-116.831, -40.9333)
  line L978 (-116.831, -40.9333) -> (-117.632, -40.9333)
  line L979 (-117.632, -40.9333) -> (-117.632, -46.7348)
  line L980 (-117.632, -46.7348) -> (-116.831, -46.7348)
  line L981 (-116.831, -46.7348) -> (-116.831, -49.8327)
  line L982 (-116.831, -49.8327) -> (-117.632, -49.8327)
  line L983 (-117.632, -49.8327) -> (-117.632, -50.833)
  line L984 (-208.12, -107.9831) -> (-222.119, -107.9831)
  line L985 (-222.119, -107.9831) -> (-222.119, -106.9826)
  line L986 (-222.119, -106.9826) -> (-222.92, -106.9826)
  line L987 (-222.92, -106.9826) -> (-222.92, -103.8834)
  line L988 (-222.92, -103.8834) -> (-222.119, -103.8834)
  line L989 (-222.119, -103.8834) -> (-222.119, -98.0834)
  line L990 (-222.119, -98.0834) -> (-222.92, -98.0834)
  line L991 (-222.92, -98.0834) -> (-222.92, -94.9828)
  line L992 (-222.92, -94.9828) -> (-222.119, -94.9828)
  line L993 (-222.119, -94.9828) -> (-222.119, -93.9838)
  line L994 (-222.119, -93.9838) -> (-208.12, -93.9838)
  line L995 (-208.12, -93.9838) -> (-208.12, -94.9828)
  line L996 (-208.12, -94.9828) -> (-207.319, -94.9828)
  line L997 (-207.319, -94.9828) -> (-207.319, -98.0834)
  line L998 (-207.319, -98.0834) -> (-208.12, -98.0834)
  line L999 (-208.12, -98.0834) -> (-208.12, -103.8834)
  line L1000 (-208.12, -103.8834) -> (-207.319, -103.8834)
  line L1001 (-207.319, -103.8834) -> (-207.319, -106.9826)
  line L1002 (-207.319, -106.9826) -> (-208.12, -106.9826)
  line L1003 (-208.12, -106.9826) -> (-208.12, -107.9831)
  line L1004 (-60.4822, -50.833) -> (-74.4815, -50.833)
  line L1005 (-74.4815, -50.833) -> (-74.4815, -49.8327)
  line L1006 (-74.4815, -49.8327) -> (-75.2809, -49.8327)
  line L1007 (-75.2809, -49.8327) -> (-75.2809, -46.7348)
  line L1008 (-75.2809, -46.7348) -> (-74.4815, -46.7348)
  line L1009 (-74.4815, -46.7348) -> (-74.4815, -40.9333)
  line L1010 (-74.4815, -40.9333) -> (-75.2809, -40.9333)
  line L1011 (-75.2809, -40.9333) -> (-75.2809, -37.8327)
  line L1012 (-75.2809, -37.8327) -> (-74.4815, -37.8327)
  line L1013 (-74.4815, -37.8327) -> (-74.4815, -36.8336)
  line L1014 (-74.4815, -36.8336) -> (-60.4822, -36.8336)
  line L1015 (-60.4822, -36.8336) -> (-60.4822, -37.8327)
  line L1016 (-60.4822, -37.8327) -> (-59.6814, -37.8327)
  line L1017 (-59.6814, -37.8327) -> (-59.6814, -40.9333)
  line L1018 (-59.6814, -40.9333) -> (-60.4822, -40.9333)
  line L1019 (-60.4822, -40.9333) -> (-60.4822, -46.7348)
  line L1020 (-60.4822, -46.7348) -> (-59.6814, -46.7348)
  line L1021 (-59.6814, -46.7348) -> (-59.6814, -49.8327)
  line L1022 (-59.6814, -49.8327) -> (-60.4822, -49.8327)
  line L1023 (-60.4822, -49.8327) -> (-60.4822, -50.833)
  line L1024 (-189.07, -107.9831) -> (-203.069, -107.9831)
  line L1025 (-203.069, -107.9831) -> (-203.069, -106.9826)
  line L1026 (-203.069, -106.9826) -> (-203.87, -106.9826)
  line L1027 (-203.87, -106.9826) -> (-203.87, -103.8834)
  line L1028 (-203.87, -103.8834) -> (-203.069, -103.8834)
  line L1029 (-203.069, -103.8834) -> (-203.069, -98.0834)
  line L1030 (-203.069, -98.0834) -> (-203.87, -98.0834)
  line L1031 (-203.87, -98.0834) -> (-203.87, -94.9828)
  line L1032 (-203.87, -94.9828) -> (-203.069, -94.9828)
  line L1033 (-203.069, -94.9828) -> (-203.069, -93.9838)
  line L1034 (-203.069, -93.9838) -> (-189.07, -93.9838)
  line L1035 (-189.07, -93.9838) -> (-189.07, -94.9828)
  line L1036 (-189.07, -94.9828) -> (-188.269, -94.9828)
  line L1037 (-188.269, -94.9828) -> (-188.269, -98.0834)
  line L1038 (-188.269, -98.0834) -> (-189.07, -98.0834)
  line L1039 (-189.07, -98.0834) -> (-189.07, -103.8834)
  line L1040 (-189.07, -103.8834) -> (-188.269, -103.8834)
  line L1041 (-188.269, -103.8834) -> (-188.269, -106.9826)
  line L1042 (-188.269, -106.9826) -> (-189.07, -106.9826)
  line L1043 (-189.07, -106.9826) -> (-189.07, -107.9831)
  line L1044 (-246.22, -107.9831) -> (-260.219, -107.9831)
  line L1045 (-260.219, -107.9831) -> (-260.219, -106.9826)
  line L1046 (-260.219, -106.9826) -> (-261.02, -106.9826)
  line L1047 (-261.02, -106.9826) -> (-261.02, -103.8834)
  line L1048 (-261.02, -103.8834) -> (-260.219, -103.8834)
  line L1049 (-260.219, -103.8834) -> (-260.219, -98.0834)
  line L1050 (-260.219, -98.0834) -> (-261.02, -98.0834)
  line L1051 (-261.02, -98.0834) -> (-261.02, -94.9828)
  line L1052 (-261.02, -94.9828) -> (-260.219, -94.9828)
  line L1053 (-260.219, -94.9828) -> (-260.219, -93.9838)
  line L1054 (-260.219, -93.9838) -> (-246.22, -93.9838)
  line L1055 (-246.22, -93.9838) -> (-246.22, -94.9828)
  line L1056 (-246.22, -94.9828) -> (-245.419, -94.9828)
  line L1057 (-245.419, -94.9828) -> (-245.419, -98.0834)
  line L1058 (-245.419, -98.0834) -> (-246.22, -98.0834)
  line L1059 (-246.22, -98.0834) -> (-246.22, -103.8834)
  line L1060 (-246.22, -103.8834) -> (-245.419, -103.8834)
  line L1061 (-245.419, -103.8834) -> (-245.419, -106.9826)
  line L1062 (-245.419, -106.9826) -> (-246.22, -106.9826)
  line L1063 (-246.22, -106.9826) -> (-246.22, -107.9831)
  line L1064 (-241.457, -69.8831) -> (-255.457, -69.8831)
  line L1065 (-255.457, -69.8831) -> (-255.457, -68.8826)
  line L1066 (-255.457, -68.8826) -> (-256.256, -68.8826)
  line L1067 (-256.256, -68.8826) -> (-256.256, -65.7834)
  line L1068 (-256.256, -65.7834) -> (-255.457, -65.7834)
  line L1069 (-255.457, -65.7834) -> (-255.457, -59.9834)
  line L1070 (-255.457, -59.9834) -> (-256.256, -59.9834)
  line L1071 (-256.256, -59.9834) -> (-256.256, -56.8828)
  line L1072 (-256.256, -56.8828) -> (-255.457, -56.8828)
  line L1073 (-255.457, -56.8828) -> (-255.457, -55.8838)
  line L1074 (-255.457, -55.8838) -> (-241.457, -55.8838)
  line L1075 (-241.457, -55.8838) -> (-241.457, -56.8828)
  line L1076 (-241.457, -56.8828) -> (-240.656, -56.8828)
  line L1077 (-240.656, -56.8828) -> (-240.656, -59.9834)
  line L1078 (-240.656, -59.9834) -> (-241.457, -59.9834)
  line L1079 (-241.457, -59.9834) -> (-241.457, -65.7834)
  line L1080 (-241.457, -65.7834) -> (-240.656, -65.7834)
  line L1081 (-240.656, -65.7834) -> (-240.656, -68.8826)
  line L1082 (-240.656, -68.8826) -> (-241.457, -68.8826)
  line L1083 (-241.457, -68.8826) -> (-241.457, -69.8831)
  line L1084 (-267.65, -50.833) -> (-281.65, -50.833)
  line L1085 (-281.65, -50.833) -> (-281.65, -49.8327)
  line L1086 (-281.65, -49.8327) -> (-282.451, -49.8327)
  line L1087 (-282.451, -49.8327) -> (-282.451, -46.7348)
  line L1088 (-282.451, -46.7348) -> (-281.65, -46.7348)
  line L1089 (-281.65, -46.7348) -> (-281.65, -46.1326)
  line L1090 (-281.65, -46.1326) -> (-283.176, -46.1326)
  line L1091 (-283.176, -46.1326) -> (-283.176, -49.3628)
  line L1092 (-283.176, -49.3628) -> (-284.9, -49.3628)
  line L1093 (-284.9, -49.3628) -> (-284.9, -50.2848)
  line L1094 (-284.9, -50.2848) -> (-288.2, -50.2848)
  line L1095 (-288.2, -50.2848) -> (-288.2, -49.3628)
  line L1096 (-288.2, -49.3628) -> (-289.925, -49.3628)
  line L1097 (-289.925, -49.3628) -> (-289.925, -46.1326)
  line L1098 (-289.925, -46.1326) -> (-290.751, -46.1326)
  line L1099 (-290.751, -46.1326) -> (-290.751, -43.3338)
  line L1100 (-290.751, -43.3338) -> (-289.925, -43.3338)
  line L1101 (-289.925, -43.3338) -> (-289.925, -37.0638)
  line L1102 (-289.925, -37.0638) -> (-288.2, -37.0638)
  line L1103 (-288.2, -37.0638) -> (-288.2, -36.0826)
  line L1104 (-288.2, -36.0826) -> (-284.9, -36.0826)
  line L1105 (-284.9, -36.0826) -> (-284.9, -37.0638)
  line L1106 (-284.9, -37.0638) -> (-283.176, -37.0638)
  line L1107 (-283.176, -37.0638) -> (-283.176, -41.5327)
  line L1108 (-283.176, -41.5327) -> (-281.65, -41.5327)
  line L1109 (-281.65, -41.5327) -> (-281.65, -40.9333)
  line L1110 (-281.65, -40.9333) -> (-282.451, -40.9333)
  line L1111 (-282.451, -40.9333) -> (-282.451, -37.8327)
  line L1112 (-282.451, -37.8327) -> (-281.65, -37.8327)
  line L1113 (-281.65, -37.8327) -> (-281.65, -36.8336)
  line L1114 (-281.65, -36.8336) -> (-267.65, -36.8336)
  line L1115 (-267.65, -36.8336) -> (-267.65, -37.8327)
  line L1116 (-267.65, -37.8327) -> (-266.849, -37.8327)
  line L1117 (-266.849, -37.8327) -> (-266.849, -40.9333)
  line L1118 (-266.849, -40.9333) -> (-267.65, -40.9333)
  line L1119 (-267.65, -40.9333) -> (-267.65, -41.5327)
  line L1120 (-267.65, -41.5327) -> (-266.126, -41.5327)
  line L1121 (-266.126, -41.5327) -> (-266.126, -37.0638)
  line L1122 (-266.126, -37.0638) -> (-264.4, -37.0638)
  line L1123 (-264.4, -37.0638) -> (-264.4, -36.0826)
  line L1124 (-264.4, -36.0826) -> (-261.101, -36.0826)
  line L1125 (-261.101, -36.0826) -> (-261.101, -37.0638)
  line L1126 (-261.101, -37.0638) -> (-259.376, -37.0638)
  line L1127 (-259.376, -37.0638) -> (-259.376, -43.3338)
  line L1128 (-259.376, -43.3338) -> (-258.55, -43.3338)
  line L1129 (-258.55, -43.3338) -> (-258.55, -46.1326)
  line L1130 (-258.55, -46.1326) -> (-259.376, -46.1326)
  line L1131 (-259.376, -46.1326) -> (-259.376, -49.3628)
  line L1132 (-259.376, -49.3628) -> (-261.101, -49.3628)
  line L1133 (-261.101, -49.3628) -> (-261.101, -50.2848)
  line L1134 (-261.101, -50.2848) -> (-264.4, -50.2848)
  line L1135 (-264.4, -50.2848) -> (-264.4, -49.3628)
  line L1136 (-264.4, -49.3628) -> (-266.126, -49.3628)
  line L1137 (-266.126, -49.3628) -> (-266.126, -46.1326)
  line L1138 (-266.126, -46.1326) -> (-267.65, -46.1326)
  line L1139 (-267.65, -46.1326) -> (-267.65, -46.7348)
  line L1140 (-267.65, -46.7348) -> (-266.849, -46.7348)
  line L1141 (-266.849, -46.7348) -> (-266.849, -49.8327)
  line L1142 (-266.849, -49.8327) -> (-267.65, -49.8327)
  line L1143 (-267.65, -49.8327) -> (-267.65, -50.833)
  line L1144 (-127.157, -69.8831) -> (-141.157, -69.8831)
  line L1145 (-141.157, -69.8831) -> (-141.157, -68.8826)
  line L1146 (-141.157, -68.8826) -> (-141.956, -68.8826)
  line L1147 (-141.956, -68.8826) -> (-141.956, -65.7834)
  line L1148 (-141.956, -65.7834) -> (-141.157, -65.7834)
  line L1149 (-141.157, -65.7834) -> (-141.157, -59.9834)
  line L1150 (-141.157, -59.9834) -> (-141.956, -59.9834)
  line L1151 (-141.956, -59.9834) -> (-141.956, -56.8828)
  line L1152 (-141.956, -56.8828) -> (-141.157, -56.8828)
  line L1153 (-141.157, -56.8828) -> (-141.157, -55.8838)
  line L1154 (-141.157, -55.8838) -> (-127.157, -55.8838)
  line L1155 (-127.157, -55.8838) -> (-127.157, -56.8828)
  line L1156 (-127.157, -56.8828) -> (-126.356, -56.8828)
  line L1157 (-126.356, -56.8828) -> (-126.356, -59.9834)
  line L1158 (-126.356, -59.9834) -> (-127.157, -59.9834)
  line L1159 (-127.157, -59.9834) -> (-127.157, -65.7834)
  line L1160 (-127.157, -65.7834) -> (-126.356, -65.7834)
  line L1161 (-126.356, -65.7834) -> (-126.356, -68.8826)
  line L1162 (-126.356, -68.8826) -> (-127.157, -68.8826)
  line L1163 (-127.157, -68.8826) -> (-127.157, -69.8831)
  line L1164 (-43.812, -31.7831) -> (-57.8128, -31.7831)
  line L1165 (-57.8128, -31.7831) -> (-57.8128, -30.7827)
  line L1166 (-57.8128, -30.7827) -> (-58.6122, -30.7827)
  line L1167 (-58.6122, -30.7827) -> (-58.6122, -27.6848)
  line L1168 (-58.6122, -27.6848) -> (-57.8128, -27.6848)
  line L1169 (-57.8128, -27.6848) -> (-57.8128, -21.8833)
  line L1170 (-57.8128, -21.8833) -> (-58.6122, -21.8833)
  line L1171 (-58.6122, -21.8833) -> (-58.6122, -18.7827)
  line L1172 (-58.6122, -18.7827) -> (-57.8128, -18.7827)
  line L1173 (-57.8128, -18.7827) -> (-57.8128, -17.7836)
  line L1174 (-57.8128, -17.7836) -> (-43.812, -17.7836)
  line L1175 (-43.812, -17.7836) -> (-43.812, -18.7827)
  line L1176 (-43.812, -18.7827) -> (-43.0128, -18.7827)
  line L1177 (-43.0128, -18.7827) -> (-43.0128, -21.8833)
  line L1178 (-43.0128, -21.8833) -> (-43.812, -21.8833)
  line L1179 (-43.812, -21.8833) -> (-43.812, -27.6848)
  line L1180 (-43.812, -27.6848) -> (-43.0128, -27.6848)
  line L1181 (-43.0128, -27.6848) -> (-43.0128, -30.7827)
  line L1182 (-43.0128, -30.7827) -> (-43.812, -30.7827)
  line L1183 (-43.812, -30.7827) -> (-43.812, -31.7831)
  line L1184 (-67.626, -31.7831) -> (-81.6253, -31.7831)
  line L1185 (-81.6253, -31.7831) -> (-81.6253, -30.7827)
  line L1186 (-81.6253, -30.7827) -> (-82.4261, -30.7827)
  line L1187 (-82.4261, -30.7827) -> (-82.4261, -27.6848)
  line L1188 (-82.4261, -27.6848) -> (-81.6253, -27.6848)
  line L1189 (-81.6253, -27.6848) -> (-81.6253, -21.8833)
  line L1190 (-81.6253, -21.8833) -> (-82.4261, -21.8833)
  line L1191 (-82.4261, -21.8833) -> (-82.4261, -18.7827)
  line L1192 (-82.4261, -18.7827) -> (-81.6253, -18.7827)
  line L1193 (-81.6253, -18.7827) -> (-81.6253, -17.7836)
  line L1194 (-81.6253, -17.7836) -> (-67.626, -17.7836)
  line L1195 (-67.626, -17.7836) -> (-67.626, -18.7827)
  line L1196 (-67.626, -18.7827) -> (-66.8252, -18.7827)
  line L1197 (-66.8252, -18.7827) -> (-66.8252, -21.8833)
  line L1198 (-66.8252, -21.8833) -> (-67.626, -21.8833)
  line L1199 (-67.626, -21.8833) -> (-67.626, -27.6848)
  line L1200 (-67.626, -27.6848) -> (-66.8252, -27.6848)
  line L1201 (-66.8252, -27.6848) -> (-66.8252, -30.7827)
  line L1202 (-66.8252, -30.7827) -> (-67.626, -30.7827)
  line L1203 (-67.626, -30.7827) -> (-67.626, -31.7831)
  line L1204 (-141.445, -88.9331) -> (-155.444, -88.9331)
  line L1205 (-155.444, -88.9331) -> (-155.444, -87.9326)
  line L1206 (-155.444, -87.9326) -> (-156.245, -87.9326)
  line L1207 (-156.245, -87.9326) -> (-156.245, -84.8334)
  line L1208 (-156.245, -84.8334) -> (-155.444, -84.8334)
  line L1209 (-155.444, -84.8334) -> (-155.444, -79.0334)
  line L1210 (-155.444, -79.0334) -> (-156.245, -79.0334)
  line L1211 (-156.245, -79.0334) -> (-156.245, -75.9328)
  line L1212 (-156.245, -75.9328) -> (-155.444, -75.9328)
  line L1213 (-155.444, -75.9328) -> (-155.444, -74.9338)
  line L1214 (-155.444, -74.9338) -> (-141.445, -74.9338)
  line L1215 (-141.445, -74.9338) -> (-141.445, -75.9328)
  line L1216 (-141.445, -75.9328) -> (-140.644, -75.9328)
  line L1217 (-140.644, -75.9328) -> (-140.644, -79.0334)
  line L1218 (-140.644, -79.0334) -> (-141.445, -79.0334)
  line L1219 (-141.445, -79.0334) -> (-141.445, -84.8334)
  line L1220 (-141.445, -84.8334) -> (-140.644, -84.8334)
  line L1221 (-140.644, -84.8334) -> (-140.644, -87.9326)